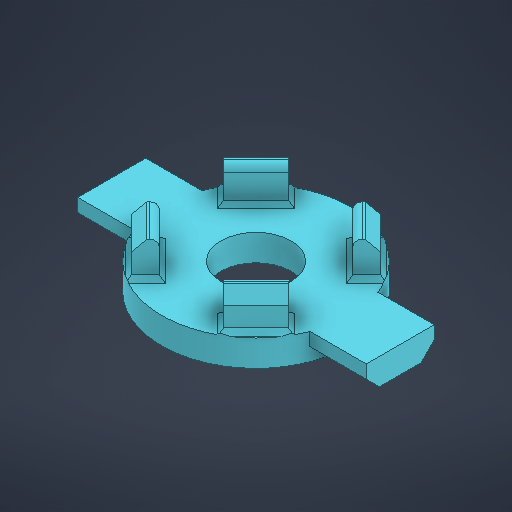
# Autodesk Inventor part: SistemLiberacion1
Saved by Autodesk Inventor 2026.1 (Build 301233000, 233)
## iProperties
Created: 2025-11-10
Part Number: SistemLiberacion1
Material: PLA
Document SubType Name: Modeling
Designer: vickh
Density: 1.3 g/cm^3
Appearance: Azul cadete
Mass: 9.17374 g
Surface Area: 43.8152 cm^2
Volume: 7.05672 cm^3
Author: vickh
## iProperties of the stored document SistemLiberacion1_3DPrint.ipt
Created: 2025-11-17
Part Number: SistemLiberacion1_3DPrint
Material: Genérico
Document SubType Name: Modeling
Designer: usuario
Density: 1 g/cm^3
Appearance: Valor por defecto
Author: usuario
Autodesk Inventor part; units mm, degrees
ref_plane "YZ Plane" through (0, 0, 0) normal (1, 0, 0) x (0, 1, 0)
ref_plane "XZ Plane" through (0, 0, 0) normal (0, 1, 0) x (-1, 0, 0)
ref_plane "XY Plane" through (0, 0, 0) normal (0, 0, 1) x (1, 0, 0)
sketch "Boceto1" plane through (0, 0, 0) normal (0, 1, 0) x (-1, 0, 0)
  line L0 (32.9046, 7.75) -> (32.9046, -7.75)
  line L1 (-32.9046, -7.75) -> (-32.9046, 7.75)
  circle A0 centre (0, 0) radius 8
  line L2 (-32.9046, 7.75) -> (-20.0546, 7.75)
  line L3 (20.0546, 7.75) -> (32.9046, 7.75)
  arc A1 (-20.0546, -7.75) -> (20.0546, -7.75) centre (0, 0) ccw
  arc A2 (20.0546, 7.75) -> (-20.0546, 7.75) centre (0, 0) ccw
  line L4 (32.9046, -7.75) -> (20.0546, -7.75)
  line L5 (-20.0546, -7.75) -> (-32.9046, -7.75)
  point P0 (-32.9046, 0)
  dimension "d55" = 16
  dimension "d58" = 21.5
  dimension "d59" = 21.5
  dimension "d61" = 15.5
  dimension "d62" = 15.5
  dimension "d77" = 12.85
  dimension "d78" = 12.85
  dimension "d79" = 65.8092
  constraints: 12 end point, 4 parallel, 4 point on circle, 3 centre point, 2 coincident, 2 horizontal, 2 perpendicular, 1 collinear, 1 midpoint
  measures "d55" diameter of A0
  measures "d58" radius of A2
  measures "d59" radius of A1
  measures "d61" distance between parallel lines of L4 L3
  measures "d62" distance of L1.start L1.end
  measures "d77" distance of L1.end L2.end
  measures "d78" distance of L3.start L0.start
  measures "d79" distance from line of L0 point (-32.905, 0)
extrude "Extrusión5" add sketch "Boceto1" against normal blind 6
sketch "Boceto5" plane through (0, 0, 0) normal (0, 1, 0) x (1, 0, 0)
  line L0 (32.9539, -32.9539) -> (-32.9539, 32.9539) construction
  line L1 (0, -51.9564) -> (0, 51.9564) construction
  line L2 (-37.6461, -37.6461) -> (37.6461, 37.6461) construction
  line L3 (-14.7432, 7.3186) -> (-7.3186, 14.7432)
  line L4 (-7.3186, 14.7432) -> (-10.5005, 17.9252)
  line L5 (-10.5005, 17.9252) -> (-17.9252, 10.5005)
  line L6 (-17.9252, 10.5005) -> (-14.7432, 7.3186)
  line L7 (-14.7432, 7.3186) -> (-10.5005, 17.9252) construction
  line L8 (-7.3186, 14.7432) -> (-17.9252, 10.5005) construction
  circle A0 centre (0, 0) radius 8 projected
  line L9 (-17.9252, -10.5005) -> (-10.5005, -17.9252)
  line L10 (-10.5005, -17.9252) -> (-7.3186, -14.7432)
  line L11 (-7.3186, -14.7432) -> (-14.7432, -7.3186)
  line L12 (-14.7432, -7.3186) -> (-17.9252, -10.5005)
  line L13 (10.5005, -17.9252) -> (17.9252, -10.5005)
  line L14 (17.9252, -10.5005) -> (14.7432, -7.3186)
  line L15 (14.7432, -7.3186) -> (7.3186, -14.7432)
  line L16 (7.3186, -14.7432) -> (10.5005, -17.9252)
  line L17 (17.9252, 10.5005) -> (10.5005, 17.9252)
  line L18 (10.5005, 17.9252) -> (7.3186, 14.7432)
  line L19 (7.3186, 14.7432) -> (14.7432, 7.3186)
  line L20 (14.7432, 7.3186) -> (17.9252, 10.5005)
  point P0 (-12.6219, 12.6219)
  dimension "d65" = 45
  dimension "d66" = 45
  dimension "d67" = 15.6
  dimension "d68" = 4.5
  dimension "d69" = 10.5
  dimension "d72" = 360
  constraints: 42 end point, 5 midpoint, 2 parallel, 2 perpendicular, 1 coincident, 1 point on line, 1 vertical, 33 other
  measures "d65" angle of L0 L1
  measures "d66" angle of L2 L1
  measures "d67" distance from line of A0.centre L3
  measures "d68" distance between parallel lines of L3 L5
  measures "d69" distance between parallel lines of L4 L6
extrude "Extrusión6" add sketch "Boceto5" along normal blind 8 contours L6 L5 L4 L3 | L12 L11 L10 L9 | L16 L15 L14 L13 | L20 L19 L18 L17
chamfer "Chaflán5" distance 3 angle 45 4 edges at (-26.4796, -6, -7.75) (-26.4796, -6, 7.75) (26.4796, -6, -7.75) (26.4796, -6, 7.75)
chamfer "Chaflán6" distance 1 angle 45 16 edges at (11.0309, 0, 11.0309) (16.3342, 0, 8.9095) (8.9095, 0, 16.3342) (14.2128, 0, 14.2128) (-11.0309, 0, 11.0309) (-8.9095, 0, 16.3342) (-16.3342, 0, 8.9095) (-14.2128, 0, 14.2128) (-14.2128, 0, -14.2128) (-8.9095, 0, -16.3342) (-11.0309, 0, -11.0309) (-16.3342, 0, -8.9095) (11.0309, 0, -11.0309) (8.9095, 0, -16.3342) (16.3342, 0, -8.9095) (14.2128, 0, -14.2128)
chamfer "Chaflán7" distance 2.5 angle 45 4 edges at (14.2128, 8, 14.2128) (14.2128, 8, -14.2128) (-14.2128, 8, -14.2128) (-14.2128, 8, 14.2128)
fillet "Empalme1" radius 1.5 4 edges at (-11.0309, 8, 11.0309) (-11.0309, 8, -11.0309) (11.0309, 8, -11.0309) (11.0309, 8, 11.0309)
